Autodesk Fusion 360 part; units mm, degrees
note: some values were not read from the file. Chosen so that the rebuilt part matches the saved one: which bodies a step acts on; which face or edge a step refers to.
(part 2 of 2)
sketch "Sketch28" plane through (0, 122.5858, 122.5858) normal (0, -0.707107, -0.707107) x (1, 0, 0) in component "Solder Reflow Hot Plate Base"
  circle A0 centre (68, -148.4924) radius 4
  line L0 (142, -169.8772) -> (142, -127.1076)
  line L1 (142, -127.1076) -> (48, -127.1076)
  line L2 (48, -127.1076) -> (48, -169.8772)
  line L3 (48, -169.8772) -> (142, -169.8772)
  line L4 (131.5, -160.2424) -> (96.5, -160.2424)
  circle A1 centre (68, -148.4924) radius 4
  line L5 (48, -148.4924) -> (142, -148.4924) construction
  line L6 (68, -148.4924) -> (68, -142.4924) construction
  line L7 (68, -142.4924) -> (78, -142.4924)
  line L8 (68, -142.4924) -> (60, -142.4924)
  line L9 (60, -142.4924) -> (60, -136.4924)
  line L10 (78, -142.4924) -> (78, -136.4924)
  line L11 (60, -136.4924) -> (78, -136.4924)
  line L12 (96.5, -160.2424) -> (96.5, -136.7424)
  line L13 (96.5, -136.7424) -> (131.5, -136.7424)
  line L14 (131.5, -136.7424) -> (131.5, -160.2424)
  dimension "d216" = 6
  dimension "d217" = 10
  dimension "d218" = 8
  dimension "d219" = 6
  dimension "d220" = 6
  constraint midpoint L2 L5.start
  constraint midpoint L0 L5.end
  constraint coincident A0.centre A1.centre
  constraint perpendicular L5 L6
  constraint perpendicular L6 L7
  constraint perpendicular L6 L8
  constraint perpendicular L8 L9
  constraint perpendicular L7 L10
  measures "d216" distance of A0.centre L6.end
  measures "d217" distance of L6.end L7.end
  measures "d218" distance of L6.end L8.end
  measures "d219" distance of L8.end L9.end
  measures "d220" distance of L7.end L10.end
extrude "Extrude30" add sketch "Sketch28" along normal blind 7 contours L7 L8 L9 L10 L11 bodies 3 in component "Solder Reflow Hot Plate Base"
sketch "Sketch29" plane through (0, 0, 0) normal (0, 0, -1) x (1, 0, 0) in component "Solder Reflow Hot Plate Base"
  line L0 (148.2, -212) -> (148.2, -210)
  line L1 (148.2, -210) -> (41.8, -210)
  line L2 (41.8, -210) -> (41.8, -212)
  line L3 (41.8, -212) -> (45, -212)
  line L4 (45, -212) -> (45, -242)
  arc A0 (45, -242) -> (48, -245) centre (48, -242) ccw
  line L5 (48, -245) -> (142, -245)
  arc A1 (142, -245) -> (145, -242) centre (142, -242) ccw
  line L6 (145, -242) -> (145, -212)
  line L7 (145, -212) -> (148.2, -212)
  line L8 (49, -210) -> (141, -210)
  line L9 (141, -210) -> (141, -241)
  line L10 (141, -241) -> (49, -241)
  line L11 (49, -241) -> (49, -210)
  dimension "d223" = 92
  dimension "d226" = 4
  dimension "d231" = 4
  constraint horizontal L8
  constraint vertical L9
  constraint horizontal L10
  constraint vertical L11
  constraint collinear L1 L8
  measures "d223" distance of L8.start L8.end
  measures "d226" distance of L6 L9
  measures "d231" distance of L5 L10
extrude "Extrude31" cut sketch "Sketch29" against normal up to surface (2 mm away) contours L1 L8 L9 L10 L11 bodies 3 in component "Solder Reflow Hot Plate Base"
fillet "Fillet6" radius 2 2 edges at (141, 241, 1) (49, 241, 1) on bodies 3 in component "Solder Reflow Hot Plate Base"
sketch "Sketch30" plane through (0, 122.5858, 122.5858) normal (0, -0.707107, -0.707107) x (1, 0, 0) in component "Solder Reflow Hot Plate Base"
  line L0 (60, -142.4924) -> (60, -136.4924)
  line L1 (60, -136.4924) -> (78, -136.4924)
  line L2 (78, -136.4924) -> (78, -142.4924)
  line L3 (78, -142.4924) -> (60, -142.4924)
  line L4 (131.5, -160.2424) -> (96.5, -160.2424)
  line L5 (96.5, -160.2424) -> (96.5, -136.7424)
  line L6 (96.5, -136.7424) -> (131.5, -136.7424)
  line L7 (131.5, -136.7424) -> (131.5, -160.2424)
  circle A0 centre (68, -148.4924) radius 4
  line L8 (142, -169.8772) -> (142, -127.1076)
  line L9 (142, -127.1076) -> (48, -127.1076)
  line L10 (48, -127.1076) -> (48, -169.8772)
  line L11 (48, -169.8772) -> (142, -169.8772)
  line L12 (96.5, -148.4924) -> (131.5, -148.4924) construction
  line L13 (114, -136.7424) -> (114, -160.2424) construction
  line L14 (134.5, -130.9924) -> (93.5, -130.9924)
  line L15 (93.5, -130.9924) -> (93.5, -165.9924)
  line L16 (93.5, -165.9924) -> (134.5, -165.9924)
  line L17 (134.5, -165.9924) -> (134.5, -130.9924)
  line L18 (134.5, -130.9924) -> (93.5, -165.9924) construction
  line L19 (93.5, -130.9924) -> (134.5, -165.9924) construction
  point P0 (114, -148.4924)
  dimension "d232" = 41
  dimension "d233" = 35
  constraint midpoint L5 L12.start
  constraint midpoint L7 L12.end
  constraint midpoint L6 L13.start
  constraint midpoint L4 L13.end
  constraint horizontal L14
  constraint perpendicular L14 L15
  constraint parallel L14 L16
  constraint parallel L15 L17
  constraint coincident L18 P0
  constraint coincident L19 P0
  constraint midpoint L13 P0
  measures "d232" distance of L15.end L16.end
  measures "d233" distance of L14.end L15.end
extrude "Extrude32" cut sketch "Sketch30" against normal blind 0.3 contours L14 L15 L16 L17 bodies 3 in component "Solder Reflow Hot Plate Base"
ref_plane "WorkPlane8" through (95, 105, 51) normal (0, 0, 1) x (1, 0, 0) in component "Solder Reflow Hot Plate Base"
sketch "Sketch32" plane through (181, 105, 51) normal (0, 0, 1) x (1, 0, 0) in component "Solder Reflow Hot Plate Base"
  line L0 (-6, 90) -> (6, 90) construction
  line L1 (-6, 102) -> (-6, 90) construction
  line L2 (-166, 90) -> (-166, 102) construction
  line L3 (-178, 90) -> (-166, 90) construction
  line L4 (6, -90) -> (-6, -90) construction
  line L5 (-6, -90) -> (-6, -102) construction
  line L6 (-166, -102) -> (-166, -90) construction
  line L7 (-166, -90) -> (-178, -90) construction
  line L8 (0, -90) -> (0, 90) construction
  line L9 (-6, 96) -> (-166, 96) construction
  line L10 (-172, 90) -> (-172, -90) construction
  line L11 (-166, -96) -> (-6, -96) construction
  circle A0 centre (-31, -96) radius 2.05
  circle A1 centre (-156, -96) radius 2.05
  circle A2 centre (-172, -65) radius 2.05
  circle A3 centre (-172, 65) radius 2.05
  circle A4 centre (-141, 96) radius 2.05
  circle A5 centre (-31, 96) radius 2.05
  circle A6 centre (0, 65) radius 2.05
  circle A7 centre (0, -65) radius 2.05
  line L12 (-146, -90) -> (-166, -90) construction
  dimension "d237" = 4.1
  dimension "d238" = 4.1
  dimension "d239" = 4.1
  dimension "d240" = 4.1
  dimension "d241" = 4.1
  dimension "d242" = 4.1
  dimension "d243" = 4.1
  dimension "d244" = 4.1
  dimension "d245" = 25
  dimension "d246" = 25
  dimension "d247" = 25
  dimension "d248" = 25
  dimension "d249" = 25
  dimension "d250" = 25
  dimension "d251" = 25
  dimension "d252" = 10
  constraint midpoint L4 L8.start
  constraint midpoint L0 L8.end
  constraint midpoint L1 L9.start
  constraint midpoint L2 L9.end
  constraint midpoint L3 L10.start
  constraint midpoint L7 L10.end
  constraint midpoint L6 L11.start
  constraint midpoint L5 L11.end
  constraint coincident L11 A0.centre
  constraint coincident L11 A1.centre
  constraint coincident L10 A2.centre
  constraint coincident L10 A3.centre
  constraint coincident L9 A4.centre
  constraint coincident L9 A5.centre
  constraint coincident L8 A6.centre
  constraint coincident L8 A7.centre
  measures "d237" diameter of A0
  measures "d238" diameter of A1
  measures "d239" diameter of A2
  measures "d240" diameter of A3
  measures "d241" diameter of A4
  measures "d242" diameter of A5
  measures "d243" diameter of A6
  measures "d244" diameter of A7
  measures "d245" distance of L4 A7.centre
  measures "d246" distance of L0 A6.centre
  measures "d247" distance of L5 A0.centre
  measures "d248" distance of L7 A2.centre
  measures "d249" distance of L3 A3.centre
  measures "d250" distance of L1 A5.centre
  measures "d251" distance of L2 A4.centre
  measures "d252" distance of L6 A1.centre
extrude "Extrude33" cut sketch "Sketch32" against normal blind 15 bodies 2 in component "Solder Reflow Hot Plate Base"
component "Solder Reflow Hot Plate Base" placed x (1, 0, 0) y (0, 1, 0) z (0, 0, 1) at (0, 0, 0)
named bodies: "Board Mount", "Sidewall", "Control Enclosure"
